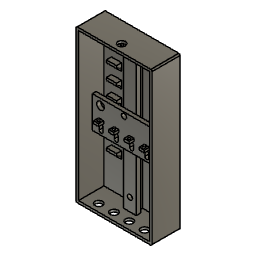
Progetto locker con bottone v3 (Autodesk Fusion 360 design; units mm, degrees)
Autodesk Fusion 360 part; units mm, degrees
note: some values were not read from the file. Set by a fixed rule: which face or edge a step refers to.
sketch "Schizzo1" plane through (0, 0, 0) normal (0, 1, 0) x (1, 0, 0) in component "Scatola di fissaggio bottone"
  line L0 (-30, -60) -> (30, -60)
  line L1 (30, -60) -> (30, 60)
  line L2 (30, 60) -> (-30, 60)
  line L3 (-30, 60) -> (-30, -60)
  point P0 (0, -60)
  point P1 (-30, 0)
  dimension "d1" = 60
  dimension "d2" = 120
  constraint horizontal L0
  constraint vertical L1
  constraint horizontal L2
  constraint vertical L3
  constraint midpoint L0 P0
  constraint midpoint L3 P1
  constraint vertical origin P0
  constraint horizontal origin P1
  measures "d1" distance of L0.start L0.end
  measures "d2" distance of L0.start L2.end
extrude "Estrusione1" add sketch "Schizzo1" along normal blind 22 makes body 1 in component "Scatola di fissaggio bottone"
shell "Svuotamento1" thickness 2 removed faces 1 at (-10, 0, 20) on bodies 1 in component "Scatola di fissaggio bottone"
ref_plane "Piano di lavoro1" through (0, 10, -58) normal (0, 0, 1) x (1, 0, 0) in component "Guida lineare"
sketch "Schizzo1 (2)" plane through (0, 12.5, -58) normal (0, 0, 1) x (1, 0, 0) in component "Guida lineare"
  line L0 (0, -26.6959) -> (0, 22.9147) construction
  line L1 (0, 0) -> (-5, 0)
  line L2 (-5, 0) -> (-5, 3.5)
  line L3 (-3.5, 5) -> (-2.5, 5)
  line L4 (-2.5, 5) -> (-2.5, 7.5)
  line L5 (28, 7.5) -> (-28, 7.5)
  line L6 (-5, 3.5) -> (-3.5, 5)
  line L7 (0, 0) -> (5, 0)
  line L8 (5, 0) -> (5, 3.5)
  line L9 (5, 3.5) -> (3.5, 5)
  line L10 (3.5, 5) -> (2.5, 5)
  line L11 (2.5, 5) -> (2.5, 7.5)
  point P0 (-5, 5)
  dimension "d7" = 2.5
  dimension "d8" = 5
  dimension "d9" = 5
  dimension "d10" = 2.5
  dimension "d11" = 1.5
  dimension "d12" = 1.5
  constraint vertical L0
  constraint coincident L1.start L0
  constraint coincident L0 L1.start
  constraint perpendicular L0 L1
  constraint perpendicular L1 L2
  constraint perpendicular L2 L3
  constraint perpendicular L3 L4
  constraint coincident L4.end L5
  constraint coincident P0 L2
  constraint coincident P0 L3
  constraint symmetric L0 L1.start L7.start
  constraint symmetric L0 L1.end L7.end
  constraint symmetric L0 L3.end L10.end
  constraint symmetric L0 L4.end L11.end
  constraint symmetric L0 L2.end L8.end
  constraint symmetric L0 L3.start L9.end
  measures "d7" distance of L3.end L4.end
  measures "d8" distance of L1.end P0
  measures "d9" distance of L1.start L1.end
  measures "d10" distance of L0 L4
  measures "d11" distance of P0 L2.end
  measures "d12" distance of P0 L3.start
extrude "Estrusione1'" add sketch "Schizzo1 (2)" along normal up to surface (116 mm away) separate body makes body 2 in component "Guida lineare"
sketch "Schizzo5" plane through (0, 0, 0) normal (0, 0, 1) x (1, 0, 0) in component "Base mobile bottone"
  line L0 (5, 16) -> (3.5, 17.5)
  line L1 (5, 12.5) -> (5, 16)
  line L2 (0, 12.5) -> (5, 12.5)
  line L3 (0, -14.1959) -> (0, 35.4147)
  line L4 (0, 12) -> (5.5, 12)
  line L5 (5.5, 12) -> (5.5, 16.2071)
  line L6 (5.5, 16.2071) -> (3.8536, 17.8536)
  line L7 (3.8536, 17.8536) -> (6.8536, 17.8536)
  line L8 (6.8536, 17.8536) -> (6.8536, 10.8536)
  line L9 (6.8536, 10.8536) -> (-0.0043, 10.8536)
  line L10 (-6.8536, 10.8536) -> (0.0043, 10.8536)
  line L11 (0, 12) -> (-5.5, 12)
  line L12 (-5.5, 12) -> (-5.5, 16.2071)
  line L13 (-5.5, 16.2071) -> (-3.8536, 17.8536)
  line L14 (-3.8536, 17.8536) -> (-6.8536, 17.8536)
  line L15 (-6.8536, 17.8536) -> (-6.8536, 10.8536)
  dimension "d135" = 0.5
  dimension "d213" = 3
  dimension "d214" = 7
  constraint perpendicular L3 L7
  constraint perpendicular L7 L8
  constraint horizontal L9
  constraint symmetric L3 L4.start L11.start
  constraint symmetric L3 L4.end L11.end
  constraint symmetric L3 L5.end L12.end
  constraint symmetric L3 L6.end L13.end
  constraint symmetric L3 L7.end L14.end
  constraint symmetric L3 L8.end L10.start
  constraint symmetric L3 L9.end L10.end
  measures "d213" distance of L6.end L7.end
  measures "d214" distance of L7.end L8.end
extrude "Estrusione2" add sketch "Schizzo5" along normal mid plane 8 separate body makes body 3 in component "Base mobile bottone"
sketch "Schizzo6" plane through (0, 10.8536, 0) normal (0, -1, 0) x (1, 0, 0) in component "Base mobile bottone"
  line L0 (0.5, 5) -> (-0.5, 5)
  line L1 (-0.5, -5) -> (0.5, -5)
  line L2 (25, -12.5) -> (-25, -12.5)
  line L3 (-25, -12.5) -> (-25, 12.5)
  line L4 (-25, 12.5) -> (25, 12.5)
  line L5 (25, 12.5) -> (25, -12.5)
  line L6 (0.8536, -4) -> (0.8536, 4)
  line L7 (0.8536, 4) -> (-0.8536, 4)
  line L8 (-0.8536, 4) -> (-0.8536, -4)
  line L9 (-0.8536, -4) -> (0.8536, -4)
  line L10 (6.8536, -4) -> (6.8536, 4)
  line L11 (6.8536, 4) -> (-6.8536, 4)
  line L12 (-6.8536, 4) -> (-6.8536, -4)
  line L13 (-6.8536, -4) -> (6.8536, -4)
  point P0 (0, -12.5)
  point P1 (25, 0)
  dimension "d31" = 50
  dimension "d32" = 25
  constraint horizontal L2
  constraint vertical L3
  constraint horizontal L4
  constraint vertical L5
  constraint midpoint L2 P0
  constraint midpoint L5 P1
  constraint horizontal origin P1
  constraint vertical origin P0
  measures "d31" distance of L2.start L2.end
  measures "d32" distance of L2.start L4.end
extrude "Estrusione3" add sketch "Schizzo6" along normal blind 3 separate body contours L2 L3 L4 L5 | L6 L7 L8 L9 L11 L13 | L6 L10 L11 L13 | L8 L11 L12 L13 makes body 4 in component "Base mobile bottone"
sketch "Schizzo3" plane through (0, 0, 60) normal (0, 0, 1) x (-1, 0, 0) in component "Scatola di fissaggio bottone"
  line L0 (30, 0) -> (-30, 0)
  line L1 (-30, 0) -> (-30, -22)
  line L2 (-30, -22) -> (30, -22)
  line L3 (30, -22) -> (30, 0)
  circle A0 centre (0, -6) radius 3
  dimension "d82" = 6
  dimension "d83" = 6
  constraint vertical origin A0.centre
  measures "d82" diameter of A0
  measures "d83" distance of L0 A0.centre
extrude "Estrusione3'" cut sketch "Schizzo3" against normal up to surface (2 mm away) contours A0 bodies 1 in component "Scatola di fissaggio bottone"
sketch "Schizzo4" plane through (0, 0, -60) normal (0, 0, -1) x (1, 0, 0) in component "Scatola di fissaggio bottone"
  line L0 (30, 0) -> (-30, 0)
  line L1 (-30, 0) -> (-30, -22)
  line L2 (-30, -22) -> (30, -22)
  line L3 (30, -22) -> (30, 0)
  circle A0 centre (-18, -6) radius 3
  line L4 (-68.094, -6) -> (66.0156, -6) construction
  line L5 (0, 54.335) -> (0, -66.5386) construction
  circle A1 centre (-6, -6) radius 3
  circle A2 centre (18, -6) radius 3
  circle A3 centre (6, -6) radius 3
  dimension "d86" = 6
  dimension "d91" = 12
  dimension "d92" = 6
  dimension "d93" = 6
  dimension "d94" = 12
  dimension "d97" = 12
  constraint perpendicular L3 L4
  constraint perpendicular L0 L5
  constraint coincident A0.centre L4
  constraint coincident L4 A1.centre
  constraint symmetric A0 L5 A2
  constraint symmetric L5 A1 A3
  measures "d86" diameter of A0
  measures "d91" distance of L1 A0.centre
  measures "d92" distance of L0 L4
  measures "d93" diameter of A1
  measures "d94" distance of A0.centre A1.centre
  measures "d97" distance of L3 A2.centre
extrude "Estrusione4" cut sketch "Schizzo4" against normal up to surface (2 mm away) contours A0 | A1 | A2 | A3 bodies 1 in component "Scatola di fissaggio bottone"
fillet "Raccordo1" radius 1 4 edges at (-30, 11, -60) (-30, 11, 60) (30, 11, 60) (30, 11, -60) on bodies 1 in component "Scatola di fissaggio bottone"
sketch "Schizzo8" plane through (0, 7.8536, 0) normal (0, -1, 0) x (1, 0, 0) in component "Base mobile bottone"
  line L0 (25, 12.5) -> (-25, 12.5)
  line L1 (-25, 12.5) -> (-25, -12.5)
  line L2 (-25, -12.5) -> (25, -12.5)
  line L3 (25, -12.5) -> (25, 12.5)
  circle A0 centre (0, 9.5) radius 2
  dimension "d101" = 4
  dimension "d102" = 3
  constraint vertical origin A0.centre
  measures "d101" diameter of A0
  measures "d102" distance of L0 A0.centre
extrude "Estrusione5" cut sketch "Schizzo8" against normal blind 3 contours A0 bodies 4 in component "Base mobile bottone"
sketch "Schizzo2" plane through (0, 7.8536, 0) normal (0, -1, 0) x (1, 0, 0)
  circle A0 centre (0, 9.5) radius 2
  line L0 (25, 12.5) -> (-25, 12.5)
  line L1 (-25, 12.5) -> (-25, -12.5)
  line L2 (-25, -12.5) -> (25, -12.5)
  line L3 (25, -12.5) -> (25, 12.5)
sketch "Schizzo3 (2)" plane through (0, 7.8536, 0) normal (0, -1, 0) x (1, 0, 0)
sketch "Schizzo4 (2)" plane through (0, 0, 0) normal (0, 0, 1) x (1, 0, 0)
  circle A0 centre (-18, 6) radius 3 construction
  circle A1 centre (-6, 6) radius 3 construction
  circle A2 centre (6, 6) radius 3 construction
  circle A3 centre (18, 6) radius 3 construction
sketch "Schizzo10" plane through (0, 7.8536, 0) normal (0, -1, 0) x (1, 0, 0) in component "Base mobile bottone"
  line L0 (-18, 0) -> (-18, -10.4085) construction
  line L1 (-6, 0) -> (-6, -9.9815) construction
  line L2 (6, 0) -> (6, -9.9815) construction
  line L3 (18, 0) -> (18, -9.9815) construction
  line L4 (-25, -12.5) -> (25, -12.5)
  line L5 (-19.5, -9.5) -> (-19.5, -6.5)
  line L6 (-16.5, -9.5) -> (-16.5, -6.5)
  arc A0 (-16.5, -6.5) -> (-19.5, -6.5) centre (-18, -6.5) ccw
  arc A1 (-19.5, -9.5) -> (-16.5, -9.5) centre (-18, -9.5) ccw
  line L7 (-12, 0.0355) -> (-12, -13.6259) construction
  arc A2 (-4.5, -6.5) -> (-7.5, -6.5) centre (-6, -6.5) ccw
  line L8 (-4.5, -9.5) -> (-4.5, -6.5)
  line L9 (-7.5, -9.5) -> (-7.5, -6.5)
  arc A3 (-7.5, -9.5) -> (-4.5, -9.5) centre (-6, -9.5) ccw
  line L10 (0, 0) -> (0, -13.6833) construction
  line L11 (16.5, -9.5) -> (16.5, -6.5)
  arc A4 (19.5, -6.5) -> (16.5, -6.5) centre (18, -6.5) ccw
  line L12 (19.5, -9.5) -> (19.5, -6.5)
  arc A5 (16.5, -9.5) -> (19.5, -9.5) centre (18, -9.5) ccw
  line L13 (4.5, -9.5) -> (4.5, -6.5)
  arc A6 (7.5, -6.5) -> (4.5, -6.5) centre (6, -6.5) ccw
  line L14 (7.5, -9.5) -> (7.5, -6.5)
  arc A7 (4.5, -9.5) -> (7.5, -9.5) centre (6, -9.5) ccw
  point P0 (-18, 0)
  point P1 (-6, 0)
  point P2 (6, 0)
  point P3 (18, 0)
  dimension "d150" = 3
  dimension "d151" = 3
  dimension "d154" = 3
  constraint coincident P0 L0.start
  constraint vertical L0
  constraint coincident P1 L1.start
  constraint vertical L1
  constraint coincident P2 L2.start
  constraint vertical L2
  constraint coincident P3 L3.start
  constraint vertical L3
  constraint coincident L0 A1.centre
  constraint tangent L5 A1
  constraint parallel L0 L6
  constraint coincident L0 A0.centre
  constraint tangent L6 A0
  constraint tangent L5 A0
  constraint equal A0 A1
  constraint perpendicular L4 L7
  constraint symmetric L5.start L7 L8.start
  constraint symmetric L5.end L7 A2.start
  constraint symmetric L6.start L7 L9.start
  constraint symmetric L6.end L7 A2.end
  constraint symmetric A0 L7 A2
  constraint symmetric A1 L7 A3
  constraint coincident L10.start origin
  constraint perpendicular L4 L10
  constraint symmetric L5.start L10 L12.start
  constraint symmetric L5.end L10 A4.start
  constraint symmetric L6.start L10 L11.start
  constraint symmetric L6.end L10 L11.end
  constraint symmetric A0 L10 A4
  constraint symmetric A1 L10 A5
  constraint symmetric A2.end L10 A6.start
  constraint symmetric A2.start L10 L13.end
  constraint symmetric A2 L10 A6
  constraint symmetric L8.start L10 L13.start
  constraint symmetric L9.start L10 L14.start
  constraint symmetric A3 L10 A7
  measures "d150" diameter of A1
  measures "d151" distance of A1.centre L4
  measures "d154" distance of A1.centre A0.centre
extrude "Estrusione7" cut sketch "Schizzo10" against normal up to surface (3 mm away) bodies 4 in component "Base mobile bottone"
sketch "Schizzo5 (2)" plane through (0, 7.8536, 0) normal (0, -1, 0) x (1, 0, 0)
  line L0 (-7.5, -9.5) -> (-7.5, -6.5)
  arc A0 (-4.5, -6.5) -> (-7.5, -6.5) centre (-6, -6.5) ccw
  line L1 (-4.5, -6.5) -> (-4.5, -9.5)
  arc A1 (-7.5, -9.5) -> (-4.5, -9.5) centre (-6, -9.5) ccw
  line L2 (4.5, -9.5) -> (4.5, -6.5)
  arc A2 (7.5, -6.5) -> (4.5, -6.5) centre (6, -6.5) ccw
  line L3 (7.5, -6.5) -> (7.5, -9.5)
  arc A3 (4.5, -9.5) -> (7.5, -9.5) centre (6, -9.5) ccw
  line L4 (-19.5, -9.5) -> (-19.5, -6.5)
  arc A4 (-16.5, -6.5) -> (-19.5, -6.5) centre (-18, -6.5) ccw
  line L5 (-16.5, -6.5) -> (-16.5, -9.5)
  arc A5 (-19.5, -9.5) -> (-16.5, -9.5) centre (-18, -9.5) ccw
  line L6 (16.5, -9.5) -> (16.5, -6.5)
  arc A6 (19.5, -6.5) -> (16.5, -6.5) centre (18, -6.5) ccw
  line L7 (19.5, -6.5) -> (19.5, -9.5)
  arc A7 (16.5, -9.5) -> (19.5, -9.5) centre (18, -9.5) ccw
  circle A8 centre (0, 9.5) radius 2
  line L8 (25, 12.5) -> (-25, 12.5)
  line L9 (-25, 12.5) -> (-25, -12.5)
  line L10 (-25, -12.5) -> (25, -12.5)
  line L11 (25, -12.5) -> (25, 12.5)
  line L12 (-1.5, 7) -> (1.5, 7)
  line L13 (1.5, 7) -> (1.5, 3)
  line L14 (1.5, 3) -> (-1.5, 3)
  line L15 (-1.5, 3) -> (-1.5, 7)
  line L16 (0, 12.5) -> (0, -12.5) construction
  line L17 (-20, -1.5) -> (-16, -1.5)
  line L18 (-16, -1.5) -> (-16, -3.5)
  line L19 (-16, -3.5) -> (-20, -3.5)
  line L20 (-20, -3.5) -> (-20, -1.5)
  line L21 (25, -12.5) -> (-25, -12.5)
  line L22 (-18, 0) -> (-18, -10.4085)
  line L23 (-6, 0) -> (-6, -9.9815)
  line L24 (6, 0) -> (6, -9.9815)
  line L25 (18, 0) -> (18, -9.9815)
  line L26 (-12, 0.0355) -> (-12, -13.6259)
  line L27 (0, 0) -> (0, -13.6833)
  line L28 (-4, -1.5) -> (-8, -1.5)
  line L29 (-4, -3.5) -> (-4, -1.5)
  line L30 (-8, -3.5) -> (-4, -3.5)
  line L31 (-8, -1.5) -> (-8, -3.5)
  line L32 (8, -1.5) -> (8, -3.5)
  line L33 (8, -3.5) -> (4, -3.5)
  line L34 (4, -3.5) -> (4, -1.5)
  line L35 (4, -1.5) -> (8, -1.5)
  line L36 (20, -3.5) -> (20, -1.5)
  line L37 (16, -3.5) -> (20, -3.5)
  line L38 (16, -1.5) -> (16, -3.5)
  line L39 (20, -1.5) -> (16, -1.5)
  dimension "d155" = 4
  dimension "d156" = 3
  dimension "d157" = 5.5
  dimension "d158" = 4
  dimension "d159" = 5
  dimension "d160" = 2
  dimension "d161" = 9
  constraint horizontal L12
  constraint vertical L13
  constraint horizontal L14
  constraint vertical L15
  constraint midpoint L8 L16.start
  constraint midpoint L10 L16.end
  constraint symmetric L13 L15 L16
  constraint horizontal L17
  constraint vertical L18
  constraint horizontal L19
  constraint vertical L20
  constraint symmetric L17.start L26 L28.start
  constraint symmetric L17.end L26 L28.end
  constraint symmetric L18.end L26 L30.start
  constraint symmetric L19.end L26 L29.start
  constraint symmetric L16 L17.start L36.end
  constraint symmetric L16 L17.end L38.start
  constraint symmetric L16 L18.end L37.start
  constraint symmetric L16 L19.end L36.start
  constraint symmetric L16 L28.start L34.end
  constraint symmetric L16 L28.end L32.start
  constraint symmetric L16 L29.start L33.end
  constraint symmetric L16 L30.start L32.end
  measures "d155" distance of L12.start L14.end
  measures "d156" distance of L13.end L14.end
  measures "d157" distance of L12 L16.start
  measures "d158" distance of L17.start L17.end
  measures "d159" distance of L9 L20
  measures "d160" distance of L17.start L19.end
  measures "d161" distance of L19 L21
extrude "Estrusione8" add sketch "Schizzo5 (2)" along normal blind 4 contours L17 L19 L20 L22 | L17 L18 L19 L22 | L23 L28 L29 L30 | L23 L28 L30 L31 | L24 L32 L33 L35 | L24 L33 L34 L35 | L25 L36 L37 L39 | L25 L37 L38 L39 bodies 4 in component "Base mobile bottone"
sketch "Schizzo6 (2)" plane through (0, 0, -3.5) normal (0, 0, -1) x (1, 0, 0)
  line L0 (-20, -7.8536) -> (-16, -7.8536)
  line L1 (-16, -7.8536) -> (-16, -3.8536)
  line L2 (-16, -3.8536) -> (-20, -3.8536)
  line L3 (-20, -3.8536) -> (-20, -7.8536)
  circle A0 centre (-18, -5.8536) radius 1
  circle A1 centre (-6, -5.8536) radius 1
  circle A2 centre (6, -5.8536) radius 1
  circle A3 centre (18, -5.8536) radius 1
  line L4 (-8, -7.8536) -> (-8, -3.8536)
  line L5 (4, -7.8536) -> (4, -3.8536)
  line L6 (16, -7.8536) -> (16, -3.8536)
  dimension "d164" = 2
  dimension "d165" = 2
  dimension "d166" = 2
  dimension "d167" = 2
  dimension "d168" = 2
  dimension "d169" = 2
  constraint equal A0 A1
  constraint equal A1 A2
  constraint equal A2 A3
  constraint horizontal A0.centre A1.centre
  constraint horizontal A1.centre A2.centre
  constraint horizontal A2.centre A3.centre
  measures "d164" diameter of A0
  measures "d165" distance of L3 A0.centre
  measures "d166" distance of L2 A0.centre
  measures "d167" distance of A1.centre L4
  measures "d168" distance of A2.centre L5
  measures "d169" distance of A3.centre L6
extrude "Estrusione9" cut sketch "Schizzo6 (2)" against normal up to surface (2 mm away) contours A0 | A1 | A2 | A3 bodies 4 in component "Base mobile bottone"
sketch "Schizzo8 (2)" plane through (0, 10.8536, 0) normal (0, 1, 0) x (-1, 0, 0)
  line L0 (7.5, -6.5) -> (7.5, -9.5)
  arc A0 (4.5, -9.5) -> (7.5, -9.5) centre (6, -9.5) ccw
  line L1 (4.5, -9.5) -> (4.5, -6.5)
  arc A1 (7.5, -6.5) -> (4.5, -6.5) centre (6, -6.5) ccw
  line L2 (-4.5, -6.5) -> (-4.5, -9.5)
  arc A2 (-7.5, -9.5) -> (-4.5, -9.5) centre (-6, -9.5) ccw
  line L3 (-7.5, -9.5) -> (-7.5, -6.5)
  arc A3 (-4.5, -6.5) -> (-7.5, -6.5) centre (-6, -6.5) ccw
  line L4 (19.5, -6.5) -> (19.5, -9.5)
  arc A4 (16.5, -9.5) -> (19.5, -9.5) centre (18, -9.5) ccw
  line L5 (16.5, -9.5) -> (16.5, -6.5)
  arc A5 (19.5, -6.5) -> (16.5, -6.5) centre (18, -6.5) ccw
  line L6 (-16.5, -6.5) -> (-16.5, -9.5)
  arc A6 (-19.5, -9.5) -> (-16.5, -9.5) centre (-18, -9.5) ccw
  line L7 (-19.5, -9.5) -> (-19.5, -6.5)
  arc A7 (-16.5, -6.5) -> (-19.5, -6.5) centre (-18, -6.5) ccw
  circle A8 centre (0, 9.5) radius 2
  line L8 (25, 12.5) -> (-25, 12.5)
  line L9 (-25, 12.5) -> (-25, -12.5)
  line L10 (-25, -12.5) -> (25, -12.5)
  line L11 (25, -12.5) -> (25, 12.5)
  line L12 (-12, 4.5) -> (-20, 4.5)
  line L13 (-20, 4.5) -> (-20, 8.5)
  line L14 (-20, 8.5) -> (-12, 8.5)
  line L15 (-12, 8.5) -> (-12, 4.5)
  dimension "d177" = 8
  dimension "d178" = 4
  dimension "d179" = 5
  dimension "d180" = 4
  constraint horizontal L12
  constraint vertical L13
  constraint horizontal L14
  constraint vertical L15
  measures "d177" distance of L12.start L12.end
  measures "d178" distance of L12.start L14.end
  measures "d179" distance of L9 L13
  measures "d180" distance of L8 L14
extrude "Estrusione11" add sketch "Schizzo8 (2)" along normal blind 5 contours L12 L13 L14 L15 bodies 4 in component "Base mobile bottone"
sketch "Schizzo9" plane through (0, 0, 4.5) normal (0, 0, -1) x (1, 0, 0)
  line L0 (20, -10.8536) -> (12, -10.8536)
  line L1 (12, -10.8536) -> (12, -15.8536)
  line L2 (12, -15.8536) -> (20, -15.8536)
  line L3 (20, -15.8536) -> (20, -10.8536)
  circle A0 centre (16, -13.8536) radius 1
  dimension "d183" = 2
  dimension "d184" = 4
  dimension "d185" = 2
  measures "d183" diameter of A0
  measures "d184" distance of L3 A0.centre
  measures "d185" distance of L2 A0.centre
extrude "Estrusione12" cut sketch "Schizzo9" against normal up to surface (4 mm away) contours A0 bodies 4 in component "Base mobile bottone"
sketch "Schizzo2 (2)" plane through (0, 12.5, 0) normal (0, -1, 0) x (1, 0, 0) in component "Guida lineare"
  line L0 (5, 58) -> (-5, 58)
  line L1 (-5, 58) -> (-5, -58)
  line L2 (-5, -58) -> (5, -58)
  line L3 (5, -58) -> (5, 58)
  circle A0 centre (0, 48) radius 2
  circle A1 centre (0, -48) radius 2
  dimension "d188" = 4
  dimension "d189" = 4
  dimension "d190" = 10
  dimension "d191" = 10
  constraint vertical origin A1.centre
  constraint vertical origin A0.centre
  measures "d188" diameter of A0
  measures "d189" diameter of A1
  measures "d190" distance of L2 A1.centre
  measures "d191" distance of L0 A0.centre
extrude "Estrusione2'" cut sketch "Schizzo2 (2)" against normal up to surface (7.5 mm away) contours A0 | A1 bodies 2 in component "Guida lineare"
sketch "Schizzo8 (3)" plane through (0, 20, 0) normal (0, -1, 0) x (1, 0, 0) in component "Scatola di fissaggio bottone"
  line L0 (-28, -58) -> (28, -58)
  line L1 (28, -58) -> (28, 58)
  line L2 (28, 58) -> (-28, 58)
  circle A0 centre (0, 48) radius 2
  circle A1 centre (0, -48) radius 2
  line L3 (-28, 58) -> (-28, -58)
extrude "Estrusione8'" cut sketch "Schizzo8 (3)" against normal up to surface (2 mm away) contours A0 | A1 bodies 1 in component "Scatola di fissaggio bottone"
sketch "Schizzo9 (2)" plane through (0, 20, 0) normal (0, -1, 0) x (1, 0, 0) in component "Scatola di fissaggio bottone"
  circle A0 centre (0, 48) radius 2
  circle A1 centre (0, -48) radius 2
  line L0 (-28, 58) -> (-28, -58)
  line L1 (-28, -58) -> (28, -58)
  line L2 (28, -58) -> (28, 58)
  line L3 (28, 58) -> (-28, 58)
  line L4 (-22, 58) -> (-14, 58)
  line L5 (-14, 58) -> (-14, -58)
  line L6 (-14, -58) -> (-22, -58)
  line L7 (-22, -58) -> (-22, 58)
  dimension "d196" = 8
  dimension "d197" = 14
  constraint horizontal L4
  constraint vertical L5
  constraint horizontal L6
  constraint vertical L7
  constraint coincident L1 L5.end
  constraint coincident L3 L4.start
  measures "d196" distance of L5 L7
  measures "d197" distance of origin L5
extrude "Estrusione9'" add sketch "Schizzo9 (2)" along normal blind 4 contours L1 L3 L4 L5 L6 L7 bodies 1 in component "Scatola di fissaggio bottone"
sketch "Schizzo11" plane through (-14, 0, 0) normal (1, 0, 0) x (0, 1, 0) in component "Scatola di fissaggio bottone"
  line L0 (20, -58) -> (20, 58)
  line L1 (20, 58) -> (16, 58)
  line L2 (16, 58) -> (16, -58)
  line L3 (16, -58) -> (20, -58)
  line L4 (16, -29) -> (16, -27)
  line L5 (20, -27) -> (20, -33)
  line L6 (16, -27) -> (20, -27)
  arc A0 (20, -33) -> (16, -29) centre (16, -33) ccw
  arc A1 (20, -21) -> (16, -17) centre (16, -21) ccw
  line L7 (16, -15) -> (20, -15)
  line L8 (16, -17) -> (16, -15)
  line L9 (20, -15) -> (20, -21)
  arc A2 (20, -9) -> (16, -5) centre (16, -9) ccw
  line L10 (16, -3) -> (20, -3)
  line L11 (16, -5) -> (16, -3)
  line L12 (20, -3) -> (20, -9)
  arc A3 (20, 3) -> (16, 7) centre (16, 3) ccw
  line L13 (16, 9) -> (20, 9)
  line L14 (16, 7) -> (16, 9)
  line L15 (20, 9) -> (20, 3)
  arc A4 (20, 15) -> (16, 19) centre (16, 15) ccw
  line L16 (16, 21) -> (20, 21)
  line L17 (16, 19) -> (16, 21)
  line L18 (20, 21) -> (20, 15)
  arc A5 (20, 27) -> (16, 31) centre (16, 27) ccw
  line L19 (16, 33) -> (20, 33)
  line L20 (16, 31) -> (16, 33)
  line L21 (20, 33) -> (20, 27)
  arc A6 (20, 39) -> (16, 43) centre (16, 39) ccw
  line L22 (16, 45) -> (20, 45)
  line L23 (16, 43) -> (16, 45)
  line L24 (20, 45) -> (20, 39)
  dimension "d200" = 2
  dimension "d201" = 25
  dimension "d204" = -12
  dimension "d205" = 10
  constraint coincident L2 A0.centre
  constraint tangent L0 A0
  constraint coincident L2 L4.start
  constraint coincident L2 L4.end
  constraint parallel L2 L4
  constraint coincident L0 L5.start
  constraint tangent L5 A0
  constraint perpendicular L5 L6
  measures "d200" distance of L4.start L4.end
  measures "d201" distance of L2.end A0.centre
extrude "Estrusione10" cut sketch "Schizzo11" against normal up to surface (8 mm away) contours L0 L2 L3 A0 | L0 L2 L6 A1 | L0 L2 L7 A2 | L0 L2 L10 A3 | L0 L2 L13 A4 | L0 L2 L16 A5 | L0 L2 L19 A6 | L0 L1 L2 L22 bodies 1 in component "Scatola di fissaggio bottone"
sketch "Schizzo10 (2)" plane through (0, 7.8536, 0) normal (0, -1, 0) x (1, 0, 0)
  line L0 (-20, -3.5) -> (-20, -1.5)
  line L1 (-20, -1.5) -> (-16, -1.5)
  line L2 (-16, -1.5) -> (-16, -3.5)
  line L3 (-16, -3.5) -> (-20, -3.5)
  line L4 (20, -1.5) -> (20, -3.5)
  line L5 (20, -3.5) -> (16, -3.5)
  line L6 (16, -3.5) -> (16, -1.5)
  line L7 (16, -1.5) -> (20, -1.5)
  line L8 (-8, -1.5) -> (-4, -1.5)
  line L9 (-4, -1.5) -> (-4, -3.5)
  line L10 (-4, -3.5) -> (-8, -3.5)
  line L11 (-8, -3.5) -> (-8, -1.5)
  line L12 (4, -1.5) -> (8, -1.5)
  line L13 (8, -1.5) -> (8, -3.5)
  line L14 (8, -3.5) -> (4, -3.5)
  line L15 (4, -3.5) -> (4, -1.5)
  line L16 (-7.5, -9.5) -> (-7.5, -6.5)
  arc A0 (-4.5, -6.5) -> (-7.5, -6.5) centre (-6, -6.5) ccw
  line L17 (-4.5, -6.5) -> (-4.5, -9.5)
  arc A1 (-7.5, -9.5) -> (-4.5, -9.5) centre (-6, -9.5) ccw
  line L18 (4.5, -9.5) -> (4.5, -6.5)
  arc A2 (7.5, -6.5) -> (4.5, -6.5) centre (6, -6.5) ccw
  line L19 (7.5, -6.5) -> (7.5, -9.5)
  arc A3 (4.5, -9.5) -> (7.5, -9.5) centre (6, -9.5) ccw
  line L20 (-19.5, -9.5) -> (-19.5, -6.5)
  arc A4 (-16.5, -6.5) -> (-19.5, -6.5) centre (-18, -6.5) ccw
  line L21 (-16.5, -6.5) -> (-16.5, -9.5)
  arc A5 (-19.5, -9.5) -> (-16.5, -9.5) centre (-18, -9.5) ccw
  line L22 (16.5, -9.5) -> (16.5, -6.5)
  arc A6 (19.5, -6.5) -> (16.5, -6.5) centre (18, -6.5) ccw
  line L23 (19.5, -6.5) -> (19.5, -9.5)
  arc A7 (16.5, -9.5) -> (19.5, -9.5) centre (18, -9.5) ccw
  circle A8 centre (0, 9.5) radius 2
  line L24 (25, 12.5) -> (-25, 12.5)
  line L25 (-25, 12.5) -> (-25, -12.5)
  line L26 (-25, -12.5) -> (25, -12.5)
  line L27 (25, -12.5) -> (25, 12.5)
  circle A9 centre (-18.5, 7.5) radius 3
  dimension "d208" = 6.5
  dimension "d209" = 6
  dimension "d210" = 5
  measures "d208" distance of L25 A9.centre
  measures "d209" diameter of A9
  measures "d210" distance of L24 A9.centre
extrude "Estrusione13" cut sketch "Schizzo10 (2)" against normal up to surface (3 mm away) contours A9 bodies 4 in component "Base mobile bottone"
component "Scatola di fissaggio bottone" placed x (1, 0, 0) y (0, 1, 0) z (0, 0, 1) at (0, 0, 0)
component "Guida lineare" placed x (1, 0, 0) y (0, 1, 0) z (0, 0, 1) at (0, 0, 0)
component "Base mobile bottone" placed x (1, 0, 0) y (0, 1, 0) z (0, 0, 1) at (0, 0, 0)
component "Bottone" placed x (1, 0, 0) y (0, 1, 0) z (0, 0, 1) at (0, 0, 0)
equation "d12 = d11"
